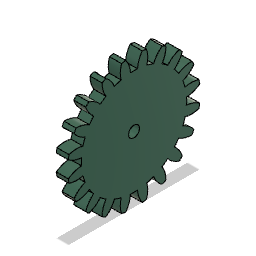
6 cm gear v5 (Autodesk Fusion 360 design; units mm, degrees)
Autodesk Fusion 360 part; units mm, degrees
sketch "Sketch1" plane through (0, 0, 0) normal (1, 0, 0) x (0, 0, -1)
  arc A0 (28.2536, 4.8202) -> (28.2536, 8.3351) centre (2.0635, 6.5776) ccw
  arc A1 (28.2536, 8.3351) -> (34.8066, 10.6867) centre (27.6511, 20.3199) ccw
  arc A2 (17.9851, 35.4827) -> (16.0896, 36.4485) centre (2.0635, 6.5776) ccw
  arc A3 (8.4852, 32.029) -> (8.2737, 38.988) centre (-3.0992, 35.1595) ccw
  arc A4 (34.8066, 10.6867) -> (34.4738, 12.7878) centre (2.0635, 6.5776) ccw
  arc A5 (6.1726, 39.3208) -> (3.8209, 32.7677) centre (15.8058, 32.1653) ccw
  arc A6 (18.8794, -13.5776) -> (24.6337, -17.4969) centre (28.2213, -6.0457) ccw
  arc A7 (16.0896, -23.2932) -> (17.9851, -22.3274) centre (2.0635, 6.5776) ccw
  arc A8 (22.2187, -10.2383) -> (24.2847, -7.3947) centre (2.0635, 6.5776) ccw
  arc A9 (3.8209, 32.7677) -> (0.306, 32.7677) centre (2.0635, 6.5776) ccw
  arc A10 (0.306, -19.6125) -> (3.8209, -19.6125) centre (2.0635, 6.5776) ccw
  arc A11 (24.6337, -17.4969) -> (26.138, -15.9926) centre (2.0635, 6.5776) ccw
  arc A12 (-13.8582, -22.3274) -> (-11.9627, -23.2932) centre (2.0635, 6.5776) ccw
  arc A13 (31.9343, -7.4485) -> (26.4286, -3.187) centre (22.1521, -14.3991) ccw
  arc A14 (6.1726, 39.3208) -> (3.8209, 32.7677) centre (15.8058, 32.1653) ccw
  arc A15 (-14.7525, -13.5776) -> (-11.9089, -15.6436) centre (2.0635, 6.5776) ccw
  arc A16 (8.2737, -25.8327) -> (8.4852, -18.8737) centre (-3.0992, -22.0043) ccw
  arc A17 (-7.7012, -17.7875) -> (-4.3583, -18.8737) centre (2.0635, 6.5776) ccw
  arc A18 (0.306, -19.6125) -> (3.8209, -19.6125) centre (2.0635, 6.5776) ccw
  arc A19 (26.4286, -3.187) -> (27.5148, 0.1559) centre (2.0635, 6.5776) ccw
  arc A20 (8.4852, -18.8737) -> (11.8281, -17.7875) centre (2.0635, 6.5776) ccw
  arc A21 (8.2737, 38.988) -> (6.1726, 39.3208) centre (2.0635, 6.5776) ccw
  arc A22 (6.1726, -26.1655) -> (8.2737, -25.8327) centre (2.0635, 6.5776) ccw
  arc A23 (8.4852, -18.8737) -> (11.8281, -17.7875) centre (2.0635, 6.5776) ccw
  arc A24 (11.8281, -17.7875) -> (16.0896, -23.2932) centre (23.0402, -13.5111) ccw
  arc A25 (30.9685, -9.344) -> (31.9343, -7.4485) centre (2.0635, 6.5776) ccw
  arc A26 (17.9851, -22.3274) -> (16.0358, -15.6436) centre (5.9857, -22.2007) ccw
  arc A27 (6.1726, -26.1655) -> (8.2737, -25.8327) centre (2.0635, 6.5776) ccw
  arc A28 (3.8209, -19.6125) -> (6.1726, -26.1655) centre (15.8058, -19.01) ccw
  arc A29 (34.4738, 0.3674) -> (34.8066, 2.4685) centre (2.0635, 6.5776) ccw
  arc A30 (34.8066, 2.4685) -> (28.2536, 4.8202) centre (27.6511, -7.1647) ccw
  arc A31 (18.8794, 26.7329) -> (16.0358, 28.7989) centre (2.0635, 6.5776) ccw
  arc A32 (-11.9089, -15.6436) -> (-13.8582, -22.3274) centre (-1.8588, -22.2007) ccw
  arc A33 (11.8281, -17.7875) -> (16.0896, -23.2932) centre (23.0402, -13.5111) ccw
  arc A34 (8.4852, 32.029) -> (8.2737, 38.988) centre (-3.0992, 35.1595) ccw
  arc A35 (16.0896, -23.2932) -> (17.9851, -22.3274) centre (2.0635, 6.5776) ccw
  arc A36 (16.0896, 36.4485) -> (11.8281, 30.9428) centre (23.0402, 26.6663) ccw
  arc A37 (16.0358, -15.6436) -> (18.8794, -13.5776) centre (2.0635, 6.5776) ccw
  arc A38 (-4.3583, -18.8737) -> (-4.1467, -25.8327) centre (7.2261, -22.0043) ccw
  arc A39 (-11.9627, -23.2932) -> (-7.7012, -17.7875) centre (-18.9133, -13.5111) ccw
  arc A40 (3.8209, -19.6125) -> (6.1726, -26.1655) centre (15.8058, -19.01) ccw
  arc A41 (11.8281, 30.9428) -> (8.4852, 32.029) centre (2.0635, 6.5776) ccw
  arc A42 (-4.1467, -25.8327) -> (-2.0457, -26.1655) centre (2.0635, 6.5776) ccw
  arc A43 (17.9851, -22.3274) -> (16.0358, -15.6436) centre (5.9857, -22.2007) ccw
  arc A44 (16.0358, -15.6436) -> (18.8794, -13.5776) centre (2.0635, 6.5776) ccw
  arc A45 (24.2847, -7.3947) -> (30.9685, -9.344) centre (30.8418, 2.6554) ccw
  arc A46 (30.9685, 22.4993) -> (24.2847, 20.55) centre (30.8418, 10.4999) ccw
  arc A47 (18.8794, 26.7329) -> (16.0358, 28.7989) centre (2.0635, 6.5776) ccw
  arc A48 (26.138, 29.1479) -> (24.6337, 30.6521) centre (2.0635, 6.5776) ccw
  arc A49 (24.2847, 20.55) -> (22.2187, 23.3936) centre (2.0635, 6.5776) ccw
  arc A50 (27.5148, 12.9994) -> (26.4286, 16.3423) centre (2.0635, 6.5776) ccw
  arc A51 (17.9851, 35.4827) -> (16.0896, 36.4485) centre (2.0635, 6.5776) ccw
  arc A52 (31.9343, 20.6038) -> (30.9685, 22.4993) centre (2.0635, 6.5776) ccw
  arc A53 (8.2737, 38.988) -> (6.1726, 39.3208) centre (2.0635, 6.5776) ccw
  arc A54 (16.0896, 36.4485) -> (11.8281, 30.9428) centre (23.0402, 26.6663) ccw
  arc A55 (24.6337, 30.6521) -> (18.8794, 26.7329) centre (28.2213, 19.201) ccw
  arc A56 (16.0358, 28.7989) -> (17.9851, 35.4827) centre (5.9857, 35.356) ccw
  arc A57 (-2.0457, -26.1655) -> (0.306, -19.6125) centre (-11.6789, -19.01) ccw
  arc A58 (16.0358, 28.7989) -> (17.9851, 35.4827) centre (5.9857, 35.356) ccw
  arc A59 (27.5148, 0.1559) -> (34.4738, 0.3674) centre (30.6454, 11.7403) ccw
  arc A60 (8.2737, -25.8327) -> (8.4852, -18.8737) centre (-3.0992, -22.0043) ccw
  arc A61 (3.8209, 32.7677) -> (0.306, 32.7677) centre (2.0635, 6.5776) ccw
  arc A62 (26.4286, 16.3423) -> (31.9343, 20.6038) centre (22.1521, 27.5544) ccw
  arc A63 (22.2187, 23.3936) -> (26.138, 29.1479) centre (14.6868, 32.7354) ccw
  arc A64 (11.8281, 30.9428) -> (8.4852, 32.029) centre (2.0635, 6.5776) ccw
  arc A65 (34.4738, 12.7878) -> (27.5148, 12.9994) centre (30.6454, 1.4149) ccw
  arc A66 (-27.8074, -7.4485) -> (-26.8416, -9.344) centre (2.0635, 6.5776) ccw
  arc A67 (30.9685, 22.4993) -> (24.2847, 20.55) centre (30.8418, 10.4999) ccw
  arc A68 (-14.7525, -13.5776) -> (-11.9089, -15.6436) centre (2.0635, 6.5776) ccw
  arc A69 (-7.7012, -17.7875) -> (-4.3583, -18.8737) centre (2.0635, 6.5776) ccw
  arc A70 (-4.3583, -18.8737) -> (-4.1467, -25.8327) centre (7.2261, -22.0043) ccw
  arc A71 (-20.5068, -17.4969) -> (-14.7525, -13.5776) centre (-24.0944, -6.0457) ccw
  arc A72 (-13.8582, -22.3274) -> (-11.9627, -23.2932) centre (2.0635, 6.5776) ccw
  arc A73 (-18.0918, -10.2383) -> (-22.0111, -15.9926) centre (-10.5599, -19.5802) ccw
  arc A74 (-30.6797, 2.4685) -> (-30.3469, 0.3674) centre (2.0635, 6.5776) ccw
  arc A75 (-27.8074, 20.6038) -> (-22.3017, 16.3423) centre (-18.0252, 27.5544) ccw
  arc A76 (-11.9089, 28.7989) -> (-14.7525, 26.7329) centre (2.0635, 6.5776) ccw
  arc A77 (24.6337, 30.6521) -> (18.8794, 26.7329) centre (28.2213, 19.201) ccw
  arc A78 (-18.0918, 23.3936) -> (-20.1578, 20.55) centre (2.0635, 6.5776) ccw
  arc A79 (-30.3469, 0.3674) -> (-23.3879, 0.1559) centre (-26.5185, 11.7403) ccw
  arc A80 (34.4738, 0.3674) -> (34.8066, 2.4685) centre (2.0635, 6.5776) ccw
  arc A81 (-7.7012, 30.9428) -> (-11.9627, 36.4485) centre (-18.9133, 26.6663) ccw
  arc A82 (34.8066, 2.4685) -> (28.2536, 4.8202) centre (27.6511, -7.1647) ccw
  arc A83 (-4.1467, 38.988) -> (-4.3583, 32.029) centre (7.2261, 35.1595) ccw
  arc A84 (-18.0918, -10.2383) -> (-22.0111, -15.9926) centre (-10.5599, -19.5802) ccw
  arc A85 (26.138, 29.1479) -> (24.6337, 30.6521) centre (2.0635, 6.5776) ccw
  arc A86 (-22.0111, -15.9926) -> (-20.5068, -17.4969) centre (2.0635, 6.5776) ccw
  arc A87 (-20.1578, -7.3947) -> (-18.0918, -10.2383) centre (2.0635, 6.5776) ccw
  arc A88 (-24.1266, 8.3351) -> (-24.1266, 4.8202) centre (2.0635, 6.5776) ccw
  arc A89 (-26.8416, -9.344) -> (-20.1578, -7.3947) centre (-26.7149, 2.6554) ccw
  arc A90 (22.2187, 23.3936) -> (26.138, 29.1479) centre (14.6868, 32.7354) ccw
  arc A91 (28.2536, 4.8202) -> (28.2536, 8.3351) centre (2.0635, 6.5776) ccw
  arc A92 (24.6337, -17.4969) -> (26.138, -15.9926) centre (2.0635, 6.5776) ccw
  arc A93 (-27.8074, -7.4485) -> (-26.8416, -9.344) centre (2.0635, 6.5776) ccw
  arc A94 (22.2187, -10.2383) -> (24.2847, -7.3947) centre (2.0635, 6.5776) ccw
  arc A95 (34.8066, 10.6867) -> (34.4738, 12.7878) centre (2.0635, 6.5776) ccw
  arc A96 (27.5148, 12.9994) -> (26.4286, 16.3423) centre (2.0635, 6.5776) ccw
  arc A97 (24.2847, 20.55) -> (22.2187, 23.3936) centre (2.0635, 6.5776) ccw
  arc A98 (28.2536, 8.3351) -> (34.8066, 10.6867) centre (27.6511, 20.3199) ccw
  arc A99 (-26.8416, 22.4993) -> (-27.8074, 20.6038) centre (2.0635, 6.5776) ccw
  arc A100 (-11.9627, -23.2932) -> (-7.7012, -17.7875) centre (-18.9133, -13.5111) ccw
  arc A101 (27.5148, 0.1559) -> (34.4738, 0.3674) centre (30.6454, 11.7403) ccw
  arc A102 (34.4738, 12.7878) -> (27.5148, 12.9994) centre (30.6454, 1.4149) ccw
  arc A103 (-22.3017, -3.187) -> (-27.8074, -7.4485) centre (-18.0252, -14.3991) ccw
  arc A104 (-20.5068, 30.6521) -> (-22.0111, 29.1479) centre (2.0635, 6.5776) ccw
  arc A105 (26.138, -15.9926) -> (22.2187, -10.2383) centre (14.6868, -19.5802) ccw
  arc A106 (26.4286, -3.187) -> (27.5148, 0.1559) centre (2.0635, 6.5776) ccw
  arc A107 (18.8794, -13.5776) -> (24.6337, -17.4969) centre (28.2213, -6.0457) ccw
  arc A108 (30.9685, -9.344) -> (31.9343, -7.4485) centre (2.0635, 6.5776) ccw
  arc A109 (31.9343, -7.4485) -> (26.4286, -3.187) centre (22.1521, -14.3991) ccw
  arc A110 (-23.3879, 0.1559) -> (-22.3017, -3.187) centre (2.0635, 6.5776) ccw
  arc A111 (26.4286, 16.3423) -> (31.9343, 20.6038) centre (22.1521, 27.5544) ccw
  arc A112 (31.9343, 20.6038) -> (30.9685, 22.4993) centre (2.0635, 6.5776) ccw
  arc A113 (-30.3469, 0.3674) -> (-23.3879, 0.1559) centre (-26.5185, 11.7403) ccw
  arc A114 (24.2847, -7.3947) -> (30.9685, -9.344) centre (30.8418, 2.6554) ccw
  arc A115 (-14.7525, 26.7329) -> (-20.5068, 30.6521) centre (-24.0944, 19.201) ccw
  arc A116 (-26.8416, -9.344) -> (-20.1578, -7.3947) centre (-26.7149, 2.6554) ccw
  arc A117 (-20.1578, -7.3947) -> (-18.0918, -10.2383) centre (2.0635, 6.5776) ccw
  arc A118 (0.306, 32.7677) -> (-2.0457, 39.3208) centre (-11.6789, 32.1653) ccw
  arc A119 (-24.1266, 4.8202) -> (-30.6797, 2.4685) centre (-23.5242, -7.1647) ccw
  arc A120 (-26.8416, 22.4993) -> (-27.8074, 20.6038) centre (2.0635, 6.5776) ccw
  arc A121 (-30.3469, 12.7878) -> (-30.6797, 10.6867) centre (2.0635, 6.5776) ccw
  arc A122 (-11.9089, -15.6436) -> (-13.8582, -22.3274) centre (-1.8588, -22.2007) ccw
  arc A123 (-4.1467, -25.8327) -> (-2.0457, -26.1655) centre (2.0635, 6.5776) ccw
  arc A124 (-23.3879, 12.9994) -> (-30.3469, 12.7878) centre (-26.5185, 1.4149) ccw
  arc A125 (-22.0111, 29.1479) -> (-18.0918, 23.3936) centre (-10.5599, 32.7354) ccw
  arc A126 (-22.3017, -3.187) -> (-27.8074, -7.4485) centre (-18.0252, -14.3991) ccw
  arc A127 (-20.5068, -17.4969) -> (-14.7525, -13.5776) centre (-24.0944, -6.0457) ccw
  arc A128 (-4.3583, 32.029) -> (-7.7012, 30.9428) centre (2.0635, 6.5776) ccw
  arc A129 (-2.0457, 39.3208) -> (-4.1467, 38.988) centre (2.0635, 6.5776) ccw
  arc A130 (-18.0918, 23.3936) -> (-20.1578, 20.55) centre (2.0635, 6.5776) ccw
  arc A131 (-23.3879, 0.1559) -> (-22.3017, -3.187) centre (2.0635, 6.5776) ccw
  arc A132 (-20.1578, 20.55) -> (-26.8416, 22.4993) centre (-26.7149, 10.4999) ccw
  arc A133 (-27.8074, 20.6038) -> (-22.3017, 16.3423) centre (-18.0252, 27.5544) ccw
  arc A134 (-2.0457, -26.1655) -> (0.306, -19.6125) centre (-11.6789, -19.01) ccw
  arc A135 (-22.0111, -15.9926) -> (-20.5068, -17.4969) centre (2.0635, 6.5776) ccw
  arc A136 (-24.1266, 8.3351) -> (-24.1266, 4.8202) centre (2.0635, 6.5776) ccw
  arc A137 (-24.1266, 4.8202) -> (-30.6797, 2.4685) centre (-23.5242, -7.1647) ccw
  arc A138 (-14.7525, 26.7329) -> (-20.5068, 30.6521) centre (-24.0944, 19.201) ccw
  arc A139 (-11.9627, 36.4485) -> (-13.8582, 35.4827) centre (2.0635, 6.5776) ccw
  arc A140 (-2.0457, 39.3208) -> (-4.1467, 38.988) centre (2.0635, 6.5776) ccw
  arc A141 (-20.1578, 20.55) -> (-26.8416, 22.4993) centre (-26.7149, 10.4999) ccw
  arc A142 (-30.3469, 12.7878) -> (-30.6797, 10.6867) centre (2.0635, 6.5776) ccw
  arc A143 (-20.5068, 30.6521) -> (-22.0111, 29.1479) centre (2.0635, 6.5776) ccw
  arc A144 (-4.1467, 38.988) -> (-4.3583, 32.029) centre (7.2261, 35.1595) ccw
  arc A145 (-11.9627, 36.4485) -> (-13.8582, 35.4827) centre (2.0635, 6.5776) ccw
  arc A146 (-30.6797, 2.4685) -> (-30.3469, 0.3674) centre (2.0635, 6.5776) ccw
  arc A147 (0.306, 32.7677) -> (-2.0457, 39.3208) centre (-11.6789, 32.1653) ccw
  arc A148 (-23.3879, 12.9994) -> (-30.3469, 12.7878) centre (-26.5185, 1.4149) ccw
  arc A149 (-13.8582, 35.4827) -> (-11.9089, 28.7989) centre (-1.8588, 35.356) ccw
  arc A150 (-13.8582, 35.4827) -> (-11.9089, 28.7989) centre (-1.8588, 35.356) ccw
  arc A151 (-22.3017, 16.3423) -> (-23.3879, 12.9994) centre (2.0635, 6.5776) ccw
  arc A152 (-4.3583, 32.029) -> (-7.7012, 30.9428) centre (2.0635, 6.5776) ccw
  arc A153 (-11.9089, 28.7989) -> (-14.7525, 26.7329) centre (2.0635, 6.5776) ccw
  arc A154 (-22.3017, 16.3423) -> (-23.3879, 12.9994) centre (2.0635, 6.5776) ccw
  arc A155 (-22.0111, 29.1479) -> (-18.0918, 23.3936) centre (-10.5599, 32.7354) ccw
  arc A156 (-7.7012, 30.9428) -> (-11.9627, 36.4485) centre (-18.9133, 26.6663) ccw
  arc A157 (-30.6797, 10.6867) -> (-24.1266, 8.3351) centre (-23.5242, 20.3199) ccw
  arc A158 (-30.6797, 10.6867) -> (-24.1266, 8.3351) centre (-23.5242, 20.3199) ccw
  arc A159 (26.138, -15.9926) -> (22.2187, -10.2383) centre (14.6868, -19.5802) ccw
  circle A160 centre (2.0635, 6.5776) radius 2.75
  dimension "d4" = 5.5
  constraint concentric A88 A160
  measures "d4" diameter of A160
extrude "Extrude1" add sketch "Sketch1" along normal blind 6
